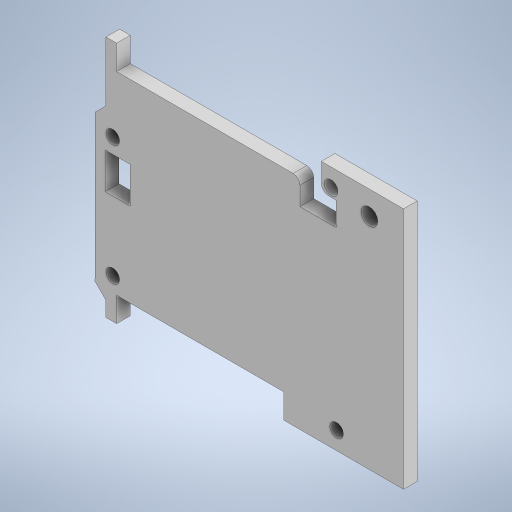
# Autodesk Inventor part: ArduinoCaseTop
Saved by Autodesk Inventor 2024 (Build 280153000, 153)
## iProperties
Created: 2023-09-08
Part Number: ArduinoCaseTop
Material: Generic
Document SubType Name: Modeling
Designer: 18179
Density: 1 g/cm^3
Appearance: Default
Autodesk Inventor part; units mm, degrees
ref_plane "YZ Plane" through (0, 0, 0) normal (1, 0, 0) x (0, 1, 0)
ref_plane "XZ Plane" through (0, 0, 0) normal (0, 1, 0) x (-1, 0, 0)
ref_plane "XY Plane" through (0, 0, 0) normal (0, 0, 1) x (1, 0, 0)
sketch "0" plane through (0, 0, 0) normal (0, 0, 1) x (1, 0, 0)
  line L0 (-4.3025, -38.4925) -> (-4.3025, 26.9125)
  arc A0 (-4.3025, 26.9125) -> (-7.4775, 30.0875) centre (-7.4775, 26.9125) ccw
  line L1 (-7.4775, 30.0875) -> (-8.7475, 30.0875)
  arc A1 (-8.7475, 30.0875) -> (-11.9225, 26.9125) centre (-8.7475, 26.9125) ccw
  line L2 (-11.9225, 26.9125) -> (-11.9225, 22.4675)
  line L3 (-11.9225, 22.4675) -> (-65.8975, 22.4675)
  line L4 (-65.8975, 22.4675) -> (-65.8975, 26.9125)
  arc A2 (-65.8975, 26.9125) -> (-69.0725, 30.0875) centre (-69.0725, 26.9125) ccw
  line L5 (-69.0725, 30.0875) -> (-70.3425, 30.0875)
  arc A3 (-70.3425, 30.0875) -> (-73.5175, 26.9125) centre (-70.3425, 26.9125) ccw
  line L6 (-73.5175, 26.9125) -> (-73.5175, 8.5836)
  line L7 (-73.5175, 8.5836) -> (-76.0575, 6.0436)
  line L8 (-76.0575, 6.0436) -> (-76.0575, -27.38)
  line L9 (-76.0575, -27.38) -> (-76.1056, -27.9894)
  line L10 (-76.1056, -27.9894) -> (-73.5175, -30.5776)
  line L11 (-73.5175, -30.5776) -> (-73.5175, -38.4925)
  arc A4 (-73.5175, -38.4925) -> (-70.3425, -41.6675) centre (-70.3425, -38.4925) ccw
  line L12 (-70.3425, -41.6675) -> (-69.0725, -41.6675)
  arc A5 (-69.0725, -41.6675) -> (-65.8975, -38.4925) centre (-69.0725, -38.4925) ccw
  line L13 (-65.8975, -38.4925) -> (-65.8975, -34.0475)
  line L14 (-65.8975, -34.0475) -> (-11.9225, -34.0475)
  line L15 (-11.9225, -34.0475) -> (-11.9225, -38.4925)
  arc A6 (-11.9225, -38.4925) -> (-8.7475, -41.6675) centre (-8.7475, -38.4925) ccw
  line L16 (-8.7475, -41.6675) -> (-7.4775, -41.6675)
  arc A7 (-7.4775, -41.6675) -> (-4.3025, -38.4925) centre (-7.4775, -38.4925) ccw
  line L17 (-5.89, 20.88) -> (-5.89, -32.46)
  line L18 (-5.89, -32.46) -> (-71.93, -32.46)
  line L19 (-71.93, -32.46) -> (-71.93, -29.92)
  line L20 (-71.93, -29.92) -> (-74.47, -27.38)
  line L21 (-74.47, -27.38) -> (-74.47, 5.386)
  line L22 (-74.47, 5.386) -> (-71.93, 7.926)
  line L23 (-71.93, 7.926) -> (-71.93, 20.88)
  line L24 (-71.93, 20.88) -> (-5.89, 20.88)
  line L25 (-48.816, 17.135) -> (-23.416, 17.135)
  line L26 (-23.416, 17.135) -> (-23.416, 19.545)
  line L27 (-23.416, 19.545) -> (-48.816, 19.545)
  line L28 (-48.816, 19.545) -> (-48.816, 17.135)
  line L29 (-46.546, 19.34) -> (-46.546, 17.34)
  line L30 (-46.546, 17.34) -> (-48.546, 17.34)
  line L31 (-48.546, 17.34) -> (-48.546, 19.34)
  line L32 (-48.546, 19.34) -> (-46.546, 19.34)
  line L33 (-44.006, 19.34) -> (-44.006, 17.34)
  line L34 (-44.006, 17.34) -> (-46.006, 17.34)
  line L35 (-46.006, 17.34) -> (-46.006, 19.34)
  line L36 (-46.006, 19.34) -> (-44.006, 19.34)
  line L37 (-41.466, 19.34) -> (-41.466, 17.34)
  line L38 (-41.466, 17.34) -> (-43.466, 17.34)
  line L39 (-43.466, 17.34) -> (-43.466, 19.34)
  line L40 (-43.466, 19.34) -> (-41.466, 19.34)
  line L41 (-38.926, 19.34) -> (-38.926, 17.34)
  line L42 (-38.926, 17.34) -> (-40.926, 17.34)
  line L43 (-40.926, 17.34) -> (-40.926, 19.34)
  line L44 (-40.926, 19.34) -> (-38.926, 19.34)
  line L45 (-36.386, 19.34) -> (-36.386, 17.34)
  line L46 (-36.386, 17.34) -> (-38.386, 17.34)
  line L47 (-38.386, 17.34) -> (-38.386, 19.34)
  line L48 (-38.386, 19.34) -> (-36.386, 19.34)
  line L49 (-33.846, 19.34) -> (-33.846, 17.34)
  line L50 (-33.846, 17.34) -> (-35.846, 17.34)
  line L51 (-35.846, 17.34) -> (-35.846, 19.34)
  line L52 (-35.846, 19.34) -> (-33.846, 19.34)
  line L53 (-31.306, 19.34) -> (-31.306, 17.34)
  line L54 (-31.306, 17.34) -> (-33.306, 17.34)
  line L55 (-33.306, 17.34) -> (-33.306, 19.34)
  line L56 (-33.306, 19.34) -> (-31.306, 19.34)
  line L57 (-28.766, 19.34) -> (-28.766, 17.34)
  line L58 (-28.766, 17.34) -> (-30.766, 17.34)
  line L59 (-30.766, 17.34) -> (-30.766, 19.34)
  line L60 (-30.766, 19.34) -> (-28.766, 19.34)
  line L61 (-26.226, 17.34) -> (-28.226, 17.34)
  line L62 (-28.226, 17.34) -> (-28.226, 19.34)
  line L63 (-28.226, 19.34) -> (-26.226, 19.34)
  line L64 (-26.226, 19.34) -> (-26.226, 17.34)
  line L65 (-25.686, 17.34) -> (-25.686, 19.34)
  line L66 (-25.686, 19.34) -> (-23.686, 19.34)
  line L67 (-23.686, 19.34) -> (-23.686, 17.34)
  line L68 (-23.686, 17.34) -> (-25.686, 17.34)
  line L69 (-20.87, 16.27) -> (-22.41, 16.27)
  arc A8 (-22.41, 16.27) -> (-22.91, 15.77) centre (-22.41, 15.77) ccw
  arc A9 (-22.91, 15.77) -> (-23.41, 16.27) centre (-23.41, 15.77) ccw
  line L70 (-23.41, 16.27) -> (-24.95, 16.27)
  arc A10 (-24.95, 16.27) -> (-25.45, 15.77) centre (-24.95, 15.77) ccw
  arc A11 (-25.45, 15.77) -> (-25.95, 16.27) centre (-25.95, 15.77) ccw
  line L71 (-25.95, 16.27) -> (-27.49, 16.27)
  arc A12 (-27.49, 16.27) -> (-27.99, 15.77) centre (-27.49, 15.77) ccw
  line L72 (-27.99, 15.77) -> (-27.99, 11.77)
  arc A13 (-27.99, 11.77) -> (-27.49, 11.27) centre (-27.49, 11.77) ccw
  line L73 (-27.49, 11.27) -> (-25.95, 11.27)
  arc A14 (-25.95, 11.27) -> (-25.45, 11.77) centre (-25.95, 11.77) ccw
  arc A15 (-25.45, 11.77) -> (-24.95, 11.27) centre (-24.95, 11.77) ccw
  line L74 (-24.95, 11.27) -> (-23.41, 11.27)
  arc A16 (-23.41, 11.27) -> (-22.91, 11.77) centre (-23.41, 11.77) ccw
  arc A17 (-22.91, 11.77) -> (-22.41, 11.27) centre (-22.41, 11.77) ccw
  line L75 (-22.41, 11.27) -> (-20.87, 11.27)
  arc A18 (-20.87, 11.27) -> (-20.37, 11.77) centre (-20.87, 11.77) ccw
  line L76 (-20.37, 11.77) -> (-20.37, 15.77)
  arc A19 (-20.37, 15.77) -> (-20.87, 16.27) centre (-20.87, 15.77) ccw
  arc A20 (-24.555, 12.6317) -> (-24.555, 12.3643) centre (-24.178, 12.498) ccw
  line L77 (-24.555, 12.6317) -> (-24.555, 12.875)
  line L78 (-24.555, 12.875) -> (-24.3117, 12.875)
  arc A21 (-24.0443, 12.875) -> (-24.3117, 12.875) centre (-24.178, 12.498) ccw
  line L79 (-24.0443, 12.875) -> (-23.805, 12.875)
  line L80 (-23.805, 12.875) -> (-23.805, 12.6425)
  arc A22 (-23.805, 12.3535) -> (-23.805, 12.6425) centre (-24.178, 12.498) ccw
  line L81 (-23.805, 12.3535) -> (-23.805, 12.125)
  line L82 (-23.805, 12.125) -> (-24.0335, 12.125)
  arc A23 (-24.3225, 12.125) -> (-24.0335, 12.125) centre (-24.178, 12.498) ccw
  line L83 (-24.3225, 12.125) -> (-24.555, 12.125)
  line L84 (-24.555, 12.125) -> (-24.555, 12.3643)
  arc A24 (-24.555, 15.1717) -> (-24.555, 14.9043) centre (-24.178, 15.038) ccw
  line L85 (-24.555, 15.1717) -> (-24.555, 15.415)
  line L86 (-24.555, 15.415) -> (-24.3117, 15.415)
  arc A25 (-24.0443, 15.415) -> (-24.3117, 15.415) centre (-24.178, 15.038) ccw
  line L87 (-24.0443, 15.415) -> (-23.805, 15.415)
  line L88 (-23.805, 15.415) -> (-23.805, 15.1825)
  arc A26 (-23.805, 14.8935) -> (-23.805, 15.1825) centre (-24.178, 15.038) ccw
  line L89 (-23.805, 14.8935) -> (-23.805, 14.665)
  line L90 (-23.805, 14.665) -> (-24.0335, 14.665)
  arc A27 (-24.3225, 14.665) -> (-24.0335, 14.665) centre (-24.178, 15.038) ccw
  line L91 (-24.3225, 14.665) -> (-24.555, 14.665)
  line L92 (-24.555, 14.665) -> (-24.555, 14.9043)
  arc A28 (-27.095, 12.6317) -> (-27.095, 12.3643) centre (-26.718, 12.498) ccw
  line L93 (-27.095, 12.6317) -> (-27.095, 12.875)
  line L94 (-27.095, 12.875) -> (-26.8517, 12.875)
  arc A29 (-26.5843, 12.875) -> (-26.8517, 12.875) centre (-26.718, 12.498) ccw
  line L95 (-26.5843, 12.875) -> (-26.345, 12.875)
  line L96 (-26.345, 12.875) -> (-26.345, 12.6425)
  arc A30 (-26.345, 12.3535) -> (-26.345, 12.6425) centre (-26.718, 12.498) ccw
  line L97 (-26.345, 12.3535) -> (-26.345, 12.125)
  line L98 (-26.345, 12.125) -> (-26.5735, 12.125)
  arc A31 (-26.8625, 12.125) -> (-26.5735, 12.125) centre (-26.718, 12.498) ccw
  line L99 (-26.8625, 12.125) -> (-27.095, 12.125)
  line L100 (-27.095, 12.125) -> (-27.095, 12.3643)
  arc A32 (-27.095, 15.1717) -> (-27.095, 14.9043) centre (-26.718, 15.038) ccw
  line L101 (-27.095, 15.1717) -> (-27.095, 15.415)
  line L102 (-27.095, 15.415) -> (-26.8517, 15.415)
  arc A33 (-26.5843, 15.415) -> (-26.8517, 15.415) centre (-26.718, 15.038) ccw
  line L103 (-26.5843, 15.415) -> (-26.345, 15.415)
  line L104 (-26.345, 15.415) -> (-26.345, 15.1825)
  arc A34 (-26.345, 14.8935) -> (-26.345, 15.1825) centre (-26.718, 15.038) ccw
  line L105 (-26.345, 14.8935) -> (-26.345, 14.665)
  line L106 (-26.345, 14.665) -> (-26.5735, 14.665)
  arc A35 (-26.8625, 14.665) -> (-26.5735, 14.665) centre (-26.718, 15.038) ccw
  line L107 (-26.8625, 14.665) -> (-27.095, 14.665)
  line L108 (-27.095, 14.665) -> (-27.095, 14.9043)
  arc A36 (-22.015, 12.6317) -> (-22.015, 12.3643) centre (-21.638, 12.498) ccw
  line L109 (-22.015, 12.6317) -> (-22.015, 12.875)
  line L110 (-22.015, 12.875) -> (-21.7717, 12.875)
  arc A37 (-21.5043, 12.875) -> (-21.7717, 12.875) centre (-21.638, 12.498) ccw
  line L111 (-21.5043, 12.875) -> (-21.265, 12.875)
  line L112 (-21.265, 12.875) -> (-21.265, 12.6425)
  arc A38 (-21.265, 12.3535) -> (-21.265, 12.6425) centre (-21.638, 12.498) ccw
  line L113 (-21.265, 12.3535) -> (-21.265, 12.125)
  line L114 (-21.265, 12.125) -> (-21.4935, 12.125)
  arc A39 (-21.7825, 12.125) -> (-21.4935, 12.125) centre (-21.638, 12.498) ccw
  line L115 (-21.7825, 12.125) -> (-22.015, 12.125)
  line L116 (-22.015, 12.125) -> (-22.015, 12.3643)
  arc A40 (-22.015, 15.1717) -> (-22.015, 14.9043) centre (-21.638, 15.038) ccw
  line L117 (-22.015, 15.1717) -> (-22.015, 15.415)
  line L118 (-22.015, 15.415) -> (-21.7717, 15.415)
  arc A41 (-21.5043, 15.415) -> (-21.7717, 15.415) centre (-21.638, 15.038) ccw
  line L119 (-21.5043, 15.415) -> (-21.265, 15.415)
  line L120 (-21.265, 15.415) -> (-21.265, 15.1825)
  arc A42 (-21.265, 14.8935) -> (-21.265, 15.1825) centre (-21.638, 15.038) ccw
  line L121 (-21.265, 14.8935) -> (-21.265, 14.665)
  line L122 (-21.265, 14.665) -> (-21.4935, 14.665)
  arc A43 (-21.7825, 14.665) -> (-21.4935, 14.665) centre (-21.638, 15.038) ccw
  line L123 (-21.7825, 14.665) -> (-22.015, 14.665)
  line L124 (-22.015, 14.665) -> (-22.015, 14.9043)
  line L125 (-70.66, 17.135) -> (-50.34, 17.135)
  line L126 (-50.34, 17.135) -> (-50.34, 19.545)
  line L127 (-50.34, 19.545) -> (-70.66, 19.545)
  line L128 (-70.66, 19.545) -> (-70.66, 17.135)
  line L129 (-68.39, 19.34) -> (-68.39, 17.34)
  line L130 (-68.39, 17.34) -> (-70.39, 17.34)
  line L131 (-70.39, 17.34) -> (-70.39, 19.34)
  line L132 (-70.39, 19.34) -> (-68.39, 19.34)
  line L133 (-65.85, 19.34) -> (-65.85, 17.34)
  line L134 (-65.85, 17.34) -> (-67.85, 17.34)
  line L135 (-67.85, 17.34) -> (-67.85, 19.34)
  line L136 (-67.85, 19.34) -> (-65.85, 19.34)
  line L137 (-63.31, 19.34) -> (-63.31, 17.34)
  line L138 (-63.31, 17.34) -> (-65.31, 17.34)
  line L139 (-65.31, 17.34) -> (-65.31, 19.34)
  line L140 (-65.31, 19.34) -> (-63.31, 19.34)
  line L141 (-60.77, 19.34) -> (-60.77, 17.34)
  line L142 (-60.77, 17.34) -> (-62.77, 17.34)
  line L143 (-62.77, 17.34) -> (-62.77, 19.34)
  line L144 (-62.77, 19.34) -> (-60.77, 19.34)
  line L145 (-58.23, 19.34) -> (-58.23, 17.34)
  line L146 (-58.23, 17.34) -> (-60.23, 17.34)
  line L147 (-60.23, 17.34) -> (-60.23, 19.34)
  line L148 (-60.23, 19.34) -> (-58.23, 19.34)
  line L149 (-55.69, 19.34) -> (-55.69, 17.34)
  line L150 (-55.69, 17.34) -> (-57.69, 17.34)
  line L151 (-57.69, 17.34) -> (-57.69, 19.34)
  line L152 (-57.69, 19.34) -> (-55.69, 19.34)
  line L153 (-53.15, 17.34) -> (-55.15, 17.34)
  line L154 (-55.15, 17.34) -> (-55.15, 19.34)
  line L155 (-55.15, 19.34) -> (-53.15, 19.34)
  line L156 (-53.15, 19.34) -> (-53.15, 17.34)
  line L157 (-52.61, 17.34) -> (-52.61, 19.34)
  line L158 (-52.61, 19.34) -> (-50.61, 19.34)
  line L159 (-50.61, 19.34) -> (-50.61, 17.34)
  line L160 (-50.61, 17.34) -> (-52.61, 17.34)
  line L161 (-73.3, -1.26) -> (-73.3, -2.8)
  arc A44 (-73.3, -2.8) -> (-72.8, -3.3) centre (-72.8, -2.8) ccw
  arc A45 (-72.8, -3.3) -> (-73.3, -3.8) centre (-72.8, -3.8) ccw
  line L162 (-73.3, -3.8) -> (-73.3, -5.34)
  arc A46 (-73.3, -5.34) -> (-72.8, -5.84) centre (-72.8, -5.34) ccw
  arc A47 (-72.8, -5.84) -> (-73.3, -6.34) centre (-72.8, -6.34) ccw
  line L163 (-73.3, -6.34) -> (-73.3, -7.88)
  arc A48 (-73.3, -7.88) -> (-72.8, -8.38) centre (-72.8, -7.88) ccw
  line L164 (-72.8, -8.38) -> (-68.8, -8.38)
  arc A49 (-68.8, -8.38) -> (-68.3, -7.88) centre (-68.8, -7.88) ccw
  line L165 (-68.3, -7.88) -> (-68.3, -6.34)
  arc A50 (-68.3, -6.34) -> (-68.8, -5.84) centre (-68.8, -6.34) ccw
  arc A51 (-68.8, -5.84) -> (-68.3, -5.34) centre (-68.8, -5.34) ccw
  line L166 (-68.3, -5.34) -> (-68.3, -3.8)
  arc A52 (-68.3, -3.8) -> (-68.8, -3.3) centre (-68.8, -3.8) ccw
  arc A53 (-68.8, -3.3) -> (-68.3, -2.8) centre (-68.8, -2.8) ccw
  line L167 (-68.3, -2.8) -> (-68.3, -1.26)
  arc A54 (-68.3, -1.26) -> (-68.8, -0.76) centre (-68.8, -1.26) ccw
  line L168 (-68.8, -0.76) -> (-72.8, -0.76)
  arc A55 (-72.8, -0.76) -> (-73.3, -1.26) centre (-72.8, -1.26) ccw
  arc A56 (-69.905, -4.4308) -> (-69.905, -4.7092) centre (-69.53, -4.57) ccw
  line L169 (-69.905, -4.4308) -> (-69.905, -4.195)
  line L170 (-69.905, -4.195) -> (-69.6692, -4.195)
  arc A57 (-69.3908, -4.195) -> (-69.6692, -4.195) centre (-69.53, -4.57) ccw
  line L171 (-69.3908, -4.195) -> (-69.155, -4.195)
  line L172 (-69.155, -4.195) -> (-69.155, -4.4308)
  arc A58 (-69.155, -4.7092) -> (-69.155, -4.4308) centre (-69.53, -4.57) ccw
  line L173 (-69.155, -4.7092) -> (-69.155, -4.945)
  line L174 (-69.155, -4.945) -> (-69.3908, -4.945)
  arc A59 (-69.6692, -4.945) -> (-69.3908, -4.945) centre (-69.53, -4.57) ccw
  line L175 (-69.6692, -4.945) -> (-69.905, -4.945)
  line L176 (-69.905, -4.945) -> (-69.905, -4.7092)
  arc A60 (-72.445, -4.4308) -> (-72.445, -4.7092) centre (-72.07, -4.57) ccw
  line L177 (-72.445, -4.4308) -> (-72.445, -4.195)
  line L178 (-72.445, -4.195) -> (-72.2092, -4.195)
  arc A61 (-71.9308, -4.195) -> (-72.2092, -4.195) centre (-72.07, -4.57) ccw
  line L179 (-71.9308, -4.195) -> (-71.695, -4.195)
  line L180 (-71.695, -4.195) -> (-71.695, -4.4308)
  arc A62 (-71.695, -4.7092) -> (-71.695, -4.4308) centre (-72.07, -4.57) ccw
  line L181 (-71.695, -4.7092) -> (-71.695, -4.945)
  line L182 (-71.695, -4.945) -> (-71.9308, -4.945)
  arc A63 (-72.2092, -4.945) -> (-71.9308, -4.945) centre (-72.07, -4.57) ccw
  line L183 (-72.2092, -4.945) -> (-72.445, -4.945)
  line L184 (-72.445, -4.945) -> (-72.445, -4.7092)
  arc A64 (-69.905, -6.9708) -> (-69.905, -7.2492) centre (-69.53, -7.11) ccw
  line L185 (-69.905, -6.9708) -> (-69.905, -6.735)
  line L186 (-69.905, -6.735) -> (-69.6692, -6.735)
  arc A65 (-69.3908, -6.735) -> (-69.6692, -6.735) centre (-69.53, -7.11) ccw
  line L187 (-69.3908, -6.735) -> (-69.155, -6.735)
  line L188 (-69.155, -6.735) -> (-69.155, -6.9708)
  arc A66 (-69.155, -7.2492) -> (-69.155, -6.9708) centre (-69.53, -7.11) ccw
  line L189 (-69.155, -7.2492) -> (-69.155, -7.485)
  line L190 (-69.155, -7.485) -> (-69.3908, -7.485)
  arc A67 (-69.6692, -7.485) -> (-69.3908, -7.485) centre (-69.53, -7.11) ccw
  line L191 (-69.6692, -7.485) -> (-69.905, -7.485)
  line L192 (-69.905, -7.485) -> (-69.905, -7.2492)
  line L193 (-72.445, -7.485) -> (-72.445, -6.735)
  line L194 (-72.445, -6.735) -> (-71.695, -6.735)
  line L195 (-71.695, -6.735) -> (-71.695, -7.485)
  line L196 (-71.695, -7.485) -> (-72.445, -7.485)
  arc A68 (-69.905, -1.8908) -> (-69.905, -2.1692) centre (-69.53, -2.03) ccw
  line L197 (-69.905, -1.8908) -> (-69.905, -1.655)
  line L198 (-69.905, -1.655) -> (-69.6692, -1.655)
  arc A69 (-69.3908, -1.655) -> (-69.6692, -1.655) centre (-69.53, -2.03) ccw
  line L199 (-69.3908, -1.655) -> (-69.155, -1.655)
  line L200 (-69.155, -1.655) -> (-69.155, -1.8908)
  arc A70 (-69.155, -2.1692) -> (-69.155, -1.8908) centre (-69.53, -2.03) ccw
  line L201 (-69.155, -2.1692) -> (-69.155, -2.405)
  line L202 (-69.155, -2.405) -> (-69.3908, -2.405)
  arc A71 (-69.6692, -2.405) -> (-69.3908, -2.405) centre (-69.53, -2.03) ccw
  line L203 (-69.6692, -2.405) -> (-69.905, -2.405)
  line L204 (-69.905, -2.405) -> (-69.905, -2.1692)
  arc A72 (-72.445, -1.8908) -> (-72.445, -2.1692) centre (-72.07, -2.03) ccw
  line L205 (-72.445, -1.8908) -> (-72.445, -1.655)
  line L206 (-72.445, -1.655) -> (-72.2092, -1.655)
  arc A73 (-71.9308, -1.655) -> (-72.2092, -1.655) centre (-72.07, -2.03) ccw
  line L207 (-71.9308, -1.655) -> (-71.695, -1.655)
  line L208 (-71.695, -1.655) -> (-71.695, -1.8908)
  arc A74 (-71.695, -2.1692) -> (-71.695, -1.8908) centre (-72.07, -2.03) ccw
  line L209 (-71.695, -2.1692) -> (-71.695, -2.405)
  line L210 (-71.695, -2.405) -> (-71.9308, -2.405)
  arc A75 (-72.2092, -2.405) -> (-71.9308, -2.405) centre (-72.07, -2.03) ccw
  line L211 (-72.2092, -2.405) -> (-72.445, -2.405)
  line L212 (-72.445, -2.405) -> (-72.445, -2.1692)
  line L213 (-70.66, -31.125) -> (-55.42, -31.125)
  line L214 (-55.42, -31.125) -> (-55.42, -28.715)
  line L215 (-55.42, -28.715) -> (-70.66, -28.715)
  line L216 (-70.66, -28.715) -> (-70.66, -31.125)
  line L217 (-68.39, -28.92) -> (-68.39, -30.92)
  line L218 (-68.39, -30.92) -> (-70.39, -30.92)
  line L219 (-70.39, -30.92) -> (-70.39, -28.92)
  line L220 (-70.39, -28.92) -> (-68.39, -28.92)
  line L221 (-65.85, -28.92) -> (-65.85, -30.92)
  line L222 (-65.85, -30.92) -> (-67.85, -30.92)
  line L223 (-67.85, -30.92) -> (-67.85, -28.92)
  line L224 (-67.85, -28.92) -> (-65.85, -28.92)
  line L225 (-63.31, -28.92) -> (-63.31, -30.92)
  line L226 (-63.31, -30.92) -> (-65.31, -30.92)
  line L227 (-65.31, -30.92) -> (-65.31, -28.92)
  line L228 (-65.31, -28.92) -> (-63.31, -28.92)
  line L229 (-60.77, -28.92) -> (-60.77, -30.92)
  line L230 (-60.77, -30.92) -> (-62.77, -30.92)
  line L231 (-62.77, -30.92) -> (-62.77, -28.92)
  line L232 (-62.77, -28.92) -> (-60.77, -28.92)
  line L233 (-58.23, -30.92) -> (-60.23, -30.92)
  line L234 (-60.23, -30.92) -> (-60.23, -28.92)
  line L235 (-60.23, -28.92) -> (-58.23, -28.92)
  line L236 (-58.23, -28.92) -> (-58.23, -30.92)
  line L237 (-57.69, -30.92) -> (-57.69, -28.92)
  line L238 (-57.69, -28.92) -> (-55.69, -28.92)
  line L239 (-55.69, -28.92) -> (-55.69, -30.92)
  line L240 (-55.69, -30.92) -> (-57.69, -30.92)
  line L241 (-52.88, -31.125) -> (-32.56, -31.125)
  line L242 (-32.56, -31.125) -> (-32.56, -28.715)
  line L243 (-32.56, -28.715) -> (-52.88, -28.715)
  line L244 (-52.88, -28.715) -> (-52.88, -31.125)
  line L245 (-50.61, -28.92) -> (-50.61, -30.92)
  line L246 (-50.61, -30.92) -> (-52.61, -30.92)
  line L247 (-52.61, -30.92) -> (-52.61, -28.92)
  line L248 (-52.61, -28.92) -> (-50.61, -28.92)
  line L249 (-48.07, -28.92) -> (-48.07, -30.92)
  line L250 (-48.07, -30.92) -> (-50.07, -30.92)
  line L251 (-50.07, -30.92) -> (-50.07, -28.92)
  line L252 (-50.07, -28.92) -> (-48.07, -28.92)
  line L253 (-45.53, -28.92) -> (-45.53, -30.92)
  line L254 (-45.53, -30.92) -> (-47.53, -30.92)
  line L255 (-47.53, -30.92) -> (-47.53, -28.92)
  line L256 (-47.53, -28.92) -> (-45.53, -28.92)
  line L257 (-42.99, -28.92) -> (-42.99, -30.92)
  line L258 (-42.99, -30.92) -> (-44.99, -30.92)
  line L259 (-44.99, -30.92) -> (-44.99, -28.92)
  line L260 (-44.99, -28.92) -> (-42.99, -28.92)
  line L261 (-40.45, -28.92) -> (-40.45, -30.92)
  line L262 (-40.45, -30.92) -> (-42.45, -30.92)
  line L263 (-42.45, -30.92) -> (-42.45, -28.92)
  line L264 (-42.45, -28.92) -> (-40.45, -28.92)
  line L265 (-37.91, -28.92) -> (-37.91, -30.92)
  line L266 (-37.91, -30.92) -> (-39.91, -30.92)
  line L267 (-39.91, -30.92) -> (-39.91, -28.92)
  line L268 (-39.91, -28.92) -> (-37.91, -28.92)
  line L269 (-35.37, -30.92) -> (-37.37, -30.92)
  line L270 (-37.37, -30.92) -> (-37.37, -28.92)
  line L271 (-37.37, -28.92) -> (-35.37, -28.92)
  line L272 (-35.37, -28.92) -> (-35.37, -30.92)
  line L273 (-34.83, -30.92) -> (-34.83, -28.92)
  line L274 (-34.83, -28.92) -> (-32.83, -28.92)
  line L275 (-32.83, -28.92) -> (-32.83, -30.92)
  line L276 (-32.83, -30.92) -> (-34.83, -30.92)
  line L277 (-74.5335, 0.814) -> (-71.93, 0.814)
  arc A76 (-71.93, 0.814) -> (-71.93, 5.386) centre (-71.93, 3.1) ccw
  line L278 (-71.93, 5.386) -> (-74.5335, 5.386)
  line L279 (-74.5335, 5.386) -> (-74.5335, 5.4123)
  line L280 (-74.5335, 5.4123) -> (-71.9935, 7.9523)
  line L281 (-71.9935, 7.9523) -> (-71.9935, 20.9435)
  line L282 (-71.9935, 20.9435) -> (-23.416, 20.9435)
  line L283 (-23.416, 20.9435) -> (-23.416, 18.34)
  arc A77 (-23.416, 18.34) -> (-18.844, 18.34) centre (-21.13, 18.34) ccw
  line L284 (-18.844, 18.34) -> (-18.844, 20.9435)
  line L285 (-18.844, 20.9435) -> (-5.8265, 20.9435)
  line L286 (-5.8265, 20.9435) -> (-5.8265, 11.12)
  line L287 (-5.8265, 11.12) -> (-5.89, 11.12)
  line L288 (-5.89, 11.12) -> (-5.89, 0)
  line L289 (-5.89, 0) -> (-5.8265, 0)
  line L290 (-5.8265, 0) -> (-5.8265, -20.285)
  line L291 (-5.8265, -20.285) -> (-5.89, -20.285)
  line L292 (-5.89, -20.285) -> (-5.89, -29.285)
  line L293 (-5.89, -29.285) -> (-5.8265, -29.285)
  line L294 (-5.8265, -29.285) -> (-5.8265, -32.5235)
  line L295 (-5.8265, -32.5235) -> (-71.9935, -32.5235)
  line L296 (-71.9935, -32.5235) -> (-71.9935, -29.9463)
  line L297 (-71.9935, -29.9463) -> (-74.5335, -27.4063)
  line L298 (-74.5335, -27.4063) -> (-74.5335, -27.126)
  line L299 (-74.5335, -27.126) -> (-71.93, -27.126)
  arc A78 (-71.93, -27.126) -> (-71.93, -22.554) centre (-71.93, -24.84) ccw
  line L300 (-71.93, -22.554) -> (-74.5335, -22.554)
  line L301 (-74.5335, -22.554) -> (-74.5335, 0.814)
  line L302 (-22.146, -29.92) -> (-22.146, -32.46)
  line L303 (-22.146, -32.46) -> (-17.574, -32.46)
  line L304 (-17.574, -32.46) -> (-17.574, -29.92)
  arc A79 (-17.574, -29.92) -> (-22.146, -29.92) centre (-19.86, -29.92) ccw
  circle A80 centre (-8.1125, -37.8575) radius 2
  circle A81 centre (-69.7075, -37.8575) radius 2
  circle A82 centre (-69.7075, 26.2775) radius 2
  circle A83 centre (-8.1125, 26.2775) radius 2
  line L305 (-47.53, -28.92) -> (-47.53, -30.92)
  circle A84 centre (-12.24, 16.943) radius 1.5
  point P0 (-20.37, 11.77)
  point P1 (-22.41, 11.27)
  point P2 (-22.91, 11.77)
  point P3 (-24.95, 11.27)
  point P4 (-27.99, 15.77)
  point P5 (-23.41, 16.27)
  point P6 (-22.91, 15.77)
  point P7 (-68.8, -0.76)
  point P8 (-68.8, -5.84)
  point P9 (-72.8, -8.38)
  point P10 (-73.5175, 26.9125)
  point P11 (-11.9225, -34.0475)
  point P12 (-74.47, 0.814)
  point P13 (-23.416, 20.88)
  point P14 (-18.844, 20.88)
  point P15 (-18.844, 18.34)
  point P16 (-20.528, 16.1347)
  point P17 (-22.1, 16.27)
  point P18 (-74.47, -27.126)
  point P19 (-74.47, -22.554)
  constraints: 612 end point, 160 point on circle, 85 centre point
extrude "Extrusion1" add sketch "0" along normal blind 3.175 contours A7 L16 A6 L15 L14 L13 A5 L12 A4 L11 L10 L9 L8 L7 L6 A3 L5 A2 L4 L3 L2 A1 L1 A0 L0 | L24 L284 L285 L286 L287 L17 | L17 L18 L304 A79 L302 L19 L20 L21 L299 A78 L300 L277 A76 L278 L22 L23 L24 L283 L27 L28 L25 L26 A77 L69 A8 A9 L70 A10 A11 L71 A12 L72 A13 L73 A14 A15 L74 A16 A17 L75 A18 L76 A19 L284 | L289 L290 L291 L17 | L24 L23 L22 L278 L279 L280 L281 L282 L283 | L293 L294 L295 L296 L297 L298 L299 L21 L20 L19 L18 L17 | L21 L300 L301 L277
sketch "Sketch3" plane through (0, 0, 3.175) normal (0, 0, 1) x (1, 0, 0)
  line L0 (-11.9225, 22.4675) -> (-65.8975, 22.4675) projected
  line L1 (-65.8975, 22.4675) -> (-76.7323, 22.4675)
  line L2 (-76.7323, 22.4675) -> (-76.7323, 33.3993)
  line L3 (-76.7323, 33.3993) -> (-65.8975, 33.3993)
  line L4 (-65.8975, 33.3993) -> (-65.8975, 22.4675)
  line L5 (-11.9225, 22.4675) -> (0, 22.4675)
  line L6 (0, 22.4675) -> (0, 30.8652)
  line L7 (0, 30.8652) -> (-11.9225, 30.8652)
  line L8 (-11.9225, 30.8652) -> (-11.9225, 22.4675)
  line L9 (-65.8975, -34.0475) -> (-11.9225, -34.0475) projected
  line L10 (-11.9225, -34.0475) -> (4.7641, -34.0475)
  line L11 (4.7641, -34.0475) -> (4.7641, -42.8261)
  line L12 (4.7641, -42.8261) -> (-11.9225, -42.8261)
  line L13 (-11.9225, -42.8261) -> (-11.9225, -34.0475)
  line L14 (-65.8975, -34.0475) -> (-80.7868, -34.0475)
  line L15 (-80.7868, -34.0475) -> (-80.7868, -44.3466)
  line L16 (-80.7868, -44.3466) -> (-65.8975, -44.3466)
  line L17 (-65.8975, -44.3466) -> (-65.8975, -34.0475)
  line L18 (-68.3, -8.38) -> (-73.3, -8.38)
  line L19 (-73.3, -8.38) -> (-73.3, -0.76)
  line L20 (-73.3, -0.76) -> (-68.3, -0.76)
  line L21 (-68.3, -0.76) -> (-68.3, -8.38)
  line L22 (-27.99, 16.27) -> (-20.37, 16.27)
  line L23 (-20.37, 16.27) -> (-20.37, 11.27)
  line L24 (-20.37, 11.27) -> (-27.99, 11.27)
  line L25 (-27.99, 11.27) -> (-27.99, 16.27)
  arc A0 (-4.3025, 26.9125) -> (-7.4775, 30.0875) centre (-7.4775, 26.9125) ccw projected
  line L26 (-7.4775, 30.0875) -> (-8.7475, 30.0875) projected
  arc A1 (-8.7475, 30.0875) -> (-11.9225, 26.9125) centre (-8.7475, 26.9125) ccw projected
  line L27 (-11.9225, 26.9125) -> (-11.9225, 22.4675) projected
  line L28 (-11.9225, 22.4675) -> (-65.8975, 22.4675) projected
  line L29 (-65.8975, 22.4675) -> (-65.8975, 26.9125) projected
  arc A2 (-65.8975, 26.9125) -> (-69.0725, 30.0875) centre (-69.0725, 26.9125) ccw projected
  line L30 (-69.0725, 30.0875) -> (-70.3425, 30.0875) projected
  arc A3 (-70.3425, 30.0875) -> (-73.5175, 26.9125) centre (-70.3425, 26.9125) ccw projected
  line L31 (-73.5175, 26.9125) -> (-73.5175, 8.5836) projected
  line L32 (-73.5175, 8.5836) -> (-76.0575, 6.0436) projected
  line L33 (-76.0575, 6.0436) -> (-76.0575, -27.38) projected
  line L34 (-76.0575, -27.38) -> (-76.1056, -27.9894) projected
  line L35 (-76.1056, -27.9894) -> (-73.5175, -30.5776) projected
  line L36 (-73.5175, -30.5776) -> (-73.5175, -38.4925) projected
  arc A4 (-73.5175, -38.4925) -> (-70.3425, -41.6675) centre (-70.3425, -38.4925) ccw projected
  line L37 (-70.3425, -41.6675) -> (-69.0725, -41.6675) projected
  arc A5 (-69.0725, -41.6675) -> (-65.8975, -38.4925) centre (-69.0725, -38.4925) ccw projected
  line L38 (-65.8975, -38.4925) -> (-65.8975, -34.0475) projected
  line L39 (-65.8975, -34.0475) -> (-11.9225, -34.0475) projected
  line L40 (-11.9225, -34.0475) -> (-11.9225, -38.4925) projected
  arc A6 (-11.9225, -38.4925) -> (-8.7475, -41.6675) centre (-8.7475, -38.4925) ccw projected
  line L41 (-8.7475, -41.6675) -> (-7.4775, -41.6675) projected
  arc A7 (-7.4775, -41.6675) -> (-4.3025, -38.4925) centre (-7.4775, -38.4925) ccw projected
  line L42 (-4.3025, -38.4925) -> (-4.3025, 26.9125) projected
  line L43 (-23.416, 18.34) -> (-23.416, 17.135) projected
  line L44 (-23.416, 17.135) -> (-48.816, 17.135) projected
  line L45 (-48.816, 17.135) -> (-48.816, 19.545) projected
  line L46 (-48.816, 19.545) -> (-23.416, 19.545) projected
  line L47 (-22.41, 16.27) -> (-22.1, 16.27) projected
  arc A8 (-20.37, 15.77) -> (-20.528, 16.1347) centre (-20.87, 15.77) ccw projected
  line L48 (-20.37, 15.77) -> (-20.37, 11.77) projected
  arc A9 (-20.87, 11.27) -> (-20.37, 11.77) centre (-20.87, 11.77) ccw projected
  line L49 (-20.87, 11.27) -> (-22.41, 11.27) projected
  arc A10 (-22.91, 11.77) -> (-22.41, 11.27) centre (-22.41, 11.77) ccw projected
  arc A11 (-23.41, 11.27) -> (-22.91, 11.77) centre (-23.41, 11.77) ccw projected
  line L50 (-23.41, 11.27) -> (-24.95, 11.27) projected
  arc A12 (-25.45, 11.77) -> (-24.95, 11.27) centre (-24.95, 11.77) ccw projected
  arc A13 (-25.95, 11.27) -> (-25.45, 11.77) centre (-25.95, 11.77) ccw projected
  line L51 (-25.95, 11.27) -> (-27.49, 11.27) projected
  arc A14 (-27.99, 11.77) -> (-27.49, 11.27) centre (-27.49, 11.77) ccw projected
  line L52 (-27.99, 11.77) -> (-27.99, 15.77) projected
  arc A15 (-27.49, 16.27) -> (-27.99, 15.77) centre (-27.49, 15.77) ccw projected
  line L53 (-27.49, 16.27) -> (-25.95, 16.27) projected
  arc A16 (-25.45, 15.77) -> (-25.95, 16.27) centre (-25.95, 15.77) ccw projected
  arc A17 (-24.95, 16.27) -> (-25.45, 15.77) centre (-24.95, 15.77) ccw projected
  line L54 (-24.95, 16.27) -> (-23.41, 16.27) projected
  arc A18 (-22.91, 15.77) -> (-23.41, 16.27) centre (-23.41, 15.77) ccw projected
  arc A19 (-22.41, 16.27) -> (-22.91, 15.77) centre (-22.41, 15.77) ccw projected
  line L55 (-70.66, 17.135) -> (-70.66, 19.545) projected
  line L56 (-70.66, 19.545) -> (-50.34, 19.545) projected
  line L57 (-50.34, 19.545) -> (-50.34, 17.135) projected
  line L58 (-50.34, 17.135) -> (-70.66, 17.135) projected
  arc A20 (-72.8, -0.76) -> (-73.3, -1.26) centre (-72.8, -1.26) ccw projected
  line L59 (-72.8, -0.76) -> (-68.8, -0.76) projected
  arc A21 (-68.3, -1.26) -> (-68.8, -0.76) centre (-68.8, -1.26) ccw projected
  line L60 (-68.3, -1.26) -> (-68.3, -2.8) projected
  arc A22 (-68.8, -3.3) -> (-68.3, -2.8) centre (-68.8, -2.8) ccw projected
  arc A23 (-68.3, -3.8) -> (-68.8, -3.3) centre (-68.8, -3.8) ccw projected
  line L61 (-68.3, -3.8) -> (-68.3, -5.34) projected
  arc A24 (-68.8, -5.84) -> (-68.3, -5.34) centre (-68.8, -5.34) ccw projected
  arc A25 (-68.3, -6.34) -> (-68.8, -5.84) centre (-68.8, -6.34) ccw projected
  line L62 (-68.3, -6.34) -> (-68.3, -7.88) projected
  arc A26 (-68.8, -8.38) -> (-68.3, -7.88) centre (-68.8, -7.88) ccw projected
  line L63 (-68.8, -8.38) -> (-72.8, -8.38) projected
  arc A27 (-73.3, -7.88) -> (-72.8, -8.38) centre (-72.8, -7.88) ccw projected
  line L64 (-73.3, -7.88) -> (-73.3, -6.34) projected
  arc A28 (-72.8, -5.84) -> (-73.3, -6.34) centre (-72.8, -6.34) ccw projected
  arc A29 (-73.3, -5.34) -> (-72.8, -5.84) centre (-72.8, -5.34) ccw projected
  line L65 (-73.3, -5.34) -> (-73.3, -3.8) projected
  arc A30 (-72.8, -3.3) -> (-73.3, -3.8) centre (-72.8, -3.8) ccw projected
  arc A31 (-73.3, -2.8) -> (-72.8, -3.3) centre (-72.8, -2.8) ccw projected
  line L66 (-73.3, -2.8) -> (-73.3, -1.26) projected
  line L67 (-70.66, -31.125) -> (-70.66, -28.715) projected
  line L68 (-70.66, -28.715) -> (-55.42, -28.715) projected
  line L69 (-55.42, -28.715) -> (-55.42, -31.125) projected
  line L70 (-55.42, -31.125) -> (-70.66, -31.125) projected
  line L71 (-52.88, -31.125) -> (-52.88, -28.715) projected
  line L72 (-52.88, -28.715) -> (-32.56, -28.715) projected
  line L73 (-32.56, -28.715) -> (-32.56, -31.125) projected
  line L74 (-32.56, -31.125) -> (-52.88, -31.125) projected
  circle A32 centre (-12.24, 16.943) radius 1.5 projected
  circle A33 centre (-8.1125, 26.2775) radius 2 projected
  circle A34 centre (-69.7075, 26.2775) radius 2 projected
  circle A35 centre (-69.7075, -37.8575) radius 2 projected
  circle A36 centre (-8.1125, -37.8575) radius 2 projected
  line L75 (-28.371, 10.889) -> (-19.989, 10.889)
  line L76 (-19.989, 10.889) -> (-19.989, 16.651)
  line L77 (-19.989, 16.651) -> (-28.371, 16.651)
  line L78 (-28.371, 16.651) -> (-28.371, 10.889)
  line L79 (-49.197, 16.754) -> (-23.035, 16.754)
  line L80 (-23.035, 16.754) -> (-23.035, 19.926)
  line L81 (-23.035, 19.926) -> (-49.197, 19.926)
  line L82 (-49.197, 19.926) -> (-49.197, 16.754)
  line L83 (-71.041, 16.754) -> (-71.041, 19.926)
  line L84 (-71.041, 19.926) -> (-49.959, 19.926)
  line L85 (-49.959, 19.926) -> (-49.959, 16.754)
  line L86 (-49.959, 16.754) -> (-71.041, 16.754)
  line L87 (-67.919, -8.761) -> (-73.681, -8.761)
  line L88 (-73.681, -8.761) -> (-73.681, -0.379)
  line L89 (-73.681, -0.379) -> (-67.919, -0.379)
  line L90 (-67.919, -0.379) -> (-67.919, -8.761)
  line L91 (-55.039, -28.334) -> (-71.041, -28.334)
  line L92 (-71.041, -28.334) -> (-71.041, -31.506)
  line L93 (-71.041, -31.506) -> (-55.039, -31.506)
  line L94 (-55.039, -31.506) -> (-55.039, -28.334)
  line L95 (-32.179, -28.334) -> (-53.261, -28.334)
  line L96 (-53.261, -28.334) -> (-53.261, -31.506)
  line L97 (-53.261, -31.506) -> (-32.179, -31.506)
  line L98 (-32.179, -31.506) -> (-32.179, -28.334)
  circle A37 centre (-12.24, 16.943) radius 1.627
  line L99 (-23.416, 20.88) -> (-18.844, 20.88) projected
  line L100 (-18.844, 20.88) -> (-18.844, 18.34) projected
  arc A38 (-20.528, 16.1347) -> (-18.844, 18.34) centre (-21.13, 18.34) ccw projected
  arc A39 (-23.416, 18.34) -> (-22.1, 16.27) centre (-21.13, 18.34) ccw projected
  line L101 (-23.416, 19.545) -> (-23.416, 20.88) projected
  point P0 (0, 0)
  dimension "d2" = 0.381
  dimension "d3" = 0.381
  dimension "d4" = 0.381
  dimension "d5" = 0.381
  dimension "d6" = 0.381
  dimension "d7" = 0.381
  dimension "d8" = 0.127
  constraints: 96 end point, 16 parallel, 8 perpendicular, 6 horizontal, 1 centre point, 18 other
  measures "d2" distance between parallel lines of L24 L75
  measures "d3" distance between parallel lines of L44 L79
  measures "d4" distance between parallel lines of L58 L86
  measures "d5" distance between parallel lines of L21 L90
  measures "d6" distance between parallel lines of L68 L91
  measures "d7" distance between parallel lines of L72 L95
  measures "d8" radial gap between concentric circles of A32 A37
extrude "Extrusion2" cut sketch "Sketch3" against normal blind 25.4 contours L8 A1 L26 A0 L42 L5 | L1 L31 A3 L30 A2 L4 | L42 A0 L26 A1 L8 L7 L6 L5 | L1 L2 L3 L4 A2 L30 A3 L31 | L42 A7 L41 A6 L13 L10 | L10 L11 L12 L13 A6 L41 A7 L42 | L17 A5 L37 A4 L36 L14 | L36 A4 L37 A5 L17 L16 L15 L14 | L18 A26 L21 | L18 A27 L19 A28 A29 A30 A31 A20 L20 A21 L21 A22 A23 A24 A25 A26 | L18 L19 A27 | A25 A24 L21 | L19 A29 A28 | A23 A22 L21 | L19 A31 A30 | A21 L20 L21 | L19 L20 A20 | L25 L24 L23 A38 L76 L75 L78 L77 A39 L22 | L22 A15 L25 | L22 A16 A17 A18 A19 L23 A38 A8 A9 L24 A10 A11 A12 A13 A14 L25 A15 | L22 A17 A16 | A14 L24 L25 | L22 A19 A18 | A13 A12 L24 | A39 L77 L76 A38 L23 L22 | A11 A10 L24 | L23 A8 A38 | A39 L43 L44 L45 L46 L101 L81 L80 | L80 L79 L82 L81 L101 L46 L45 L44 L43 A39 | A9 L23 L24 | L55 L56 L57 L58 | L67 L68 L69 L70 | L71 L72 L73 L74 | A32 | A33 | A34 | A35 | A36 | L83 L84 L85 L86 | L87 L88 L89 L90 | L94 L93 L92 L91 | L98 L97 L96 L95 | A37
sketch "Sketch4" plane through (0, 0, 3.175) normal (0, 0, 1) x (1, 0, 0)
  arc A0 (-19.989, 16.3591) -> (-18.844, 18.34) centre (-21.13, 18.34) ccw projected
  circle A1 centre (-21.13, 18.34) radius 1.5875
  arc A2 (-17.574, -29.92) -> (-22.146, -29.92) centre (-19.86, -29.92) ccw projected
  circle A3 centre (-19.86, -29.92) radius 1.5875
  arc A4 (-71.93, -27.126) -> (-71.93, -22.554) centre (-71.93, -24.84) ccw projected
  circle A5 centre (-71.93, -24.84) radius 1.5875
  arc A6 (-71.93, 0.814) -> (-71.93, 5.386) centre (-71.93, 3.1) ccw projected
  circle A7 centre (-71.93, 3.1) radius 1.5875
  line L0 (-73.5175, -34.0475) -> (-4.3025, -34.0475) projected
  line L1 (-4.3025, -34.0475) -> (-4.3025, 22.4675) projected
  line L2 (-4.3025, 22.4675) -> (-73.5175, 22.4675) projected
  line L3 (-73.5175, 22.4675) -> (-73.5175, 8.5836) projected
  line L4 (-73.5175, 8.5836) -> (-76.0575, 6.0436) projected
  line L5 (-76.0575, 6.0436) -> (-76.0575, -27.38) projected
  line L6 (-76.0575, -27.38) -> (-76.1056, -27.9894) projected
  line L7 (-76.1056, -27.9894) -> (-73.5175, -30.5776) projected
  line L8 (-73.5175, -30.5776) -> (-73.5175, -34.0475) projected
  line L9 (-28.371, 16.651) -> (-22.6705, 16.651) projected
  arc A8 (-23.035, 17.0764) -> (-22.6705, 16.651) centre (-21.13, 18.34) ccw projected
  line L10 (-23.035, 17.0764) -> (-23.035, 16.754) projected
  line L11 (-23.035, 16.754) -> (-49.197, 16.754) projected
  line L12 (-49.197, 16.754) -> (-49.197, 19.926) projected
  line L13 (-49.197, 19.926) -> (-23.416, 19.926) projected
  line L14 (-23.416, 19.926) -> (-23.416, 20.88) projected
  line L15 (-23.416, 20.88) -> (-18.844, 20.88) projected
  line L16 (-18.844, 20.88) -> (-18.844, 18.34) projected
  arc A9 (-19.989, 16.3591) -> (-18.844, 18.34) centre (-21.13, 18.34) ccw projected
  line L17 (-19.989, 16.3591) -> (-19.989, 10.889) projected
  line L18 (-19.989, 10.889) -> (-28.371, 10.889) projected
  line L19 (-28.371, 10.889) -> (-28.371, 16.651) projected
  line L20 (-32.179, -31.506) -> (-53.261, -31.506) projected
  line L21 (-53.261, -31.506) -> (-53.261, -28.334) projected
  line L22 (-53.261, -28.334) -> (-32.179, -28.334) projected
  line L23 (-32.179, -28.334) -> (-32.179, -31.506) projected
  circle A10 centre (-12.24, 16.943) radius 1.627 projected
  line L24 (-71.041, 19.926) -> (-49.959, 19.926) projected
  line L25 (-49.959, 19.926) -> (-49.959, 16.754) projected
  line L26 (-49.959, 16.754) -> (-71.041, 16.754) projected
  line L27 (-71.041, 16.754) -> (-71.041, 19.926) projected
  line L28 (-55.039, -31.506) -> (-71.041, -31.506) projected
  line L29 (-71.041, -31.506) -> (-71.041, -28.334) projected
  line L30 (-71.041, -28.334) -> (-55.039, -28.334) projected
  line L31 (-55.039, -28.334) -> (-55.039, -31.506) projected
  line L32 (-73.681, -8.761) -> (-73.681, -0.379) projected
  line L33 (-73.681, -0.379) -> (-67.919, -0.379) projected
  line L34 (-67.919, -0.379) -> (-67.919, -8.761) projected
  line L35 (-67.919, -8.761) -> (-73.681, -8.761) projected
  line L36 (-17.574, -32.46) -> (-22.146, -32.46) projected
  line L37 (-22.146, -32.46) -> (-22.146, -29.92) projected
  arc A11 (-17.574, -29.92) -> (-22.146, -29.92) centre (-19.86, -29.92) ccw projected
  line L38 (-17.574, -29.92) -> (-17.574, -32.46) projected
  line L39 (-74.47, 5.386) -> (-71.93, 5.386) projected
  arc A12 (-71.93, 0.814) -> (-71.93, 5.386) centre (-71.93, 3.1) ccw projected
  line L40 (-71.93, 0.814) -> (-74.47, 0.814) projected
  line L41 (-74.47, 0.814) -> (-74.47, 5.386) projected
  line L42 (-74.47, -27.126) -> (-74.47, -22.554) projected
  line L43 (-74.47, -22.554) -> (-71.93, -22.554) projected
  arc A13 (-71.93, -27.126) -> (-71.93, -22.554) centre (-71.93, -24.84) ccw projected
  line L44 (-71.93, -27.126) -> (-74.47, -27.126) projected
  line L45 (-22.6705, 16.651) -> (-19.989, 16.651)
  line L46 (-19.989, 16.651) -> (-19.989, 16.3591)
  line L47 (-19.989, 16.3591) -> (-22.6705, 16.651)
  line L48 (-23.035, 17.0764) -> (-23.416, 19.926)
  line L49 (-23.416, 19.926) -> (-23.035, 16.754)
  point P0 (0, 0)
  point P1 (-22.146, -29.92)
  point P2 (-71.93, 5.386)
  point P3 (-71.93, 0.814)
  dimension "d11" = 3.175
  dimension "d12" = 3.175
  dimension "d13" = 3.175
  dimension "d14" = 3.175
  constraints: 10 end point, 4 centre point, 4 coincident, 1 horizontal, 1 perpendicular
  measures "d11" diameter of A1
  measures "d12" diameter of A3
  measures "d13" diameter of A5
  measures "d14" diameter of A7
extrude "Extrusion3" add sketch "Sketch4" against normal blind 3.175 contours L46 L45 A8 L48 L14 L15 L16 A0 | L47 L45 L46 | L10 L49 L48 | L38 L36 L37 A2 | L44 L42 L43 A4 | L40 L41 L39 A6
sketch "Sketch6" plane through (0, 0, 3.175) normal (0, 0, 1) x (1, 0, 0)
  line L0 (-49.197, 19.926) -> (-23.416, 19.926) projected
  line L1 (-23.416, 19.926) -> (-23.416, 16.754)
  line L2 (-49.197, 16.754) -> (-23.035, 16.754) projected
  line L3 (-28.371, 16.651) -> (-22.6705, 16.651) projected
  line L4 (-23.416, 16.651) -> (-23.416, 16.3591)
  line L5 (-19.989, 16.3591) -> (-19.989, 10.889) projected
  line L6 (-23.416, 16.3591) -> (-19.989, 16.3591)
  circle A0 centre (-71.93, -24.84) radius 1.5875 projected
  circle A1 centre (-71.93, 3.1) radius 1.5875 projected
  circle A2 centre (-19.86, -29.92) radius 1.5875 projected
  line L7 (-19.989, 16.3591) -> (-19.989, 10.889) projected
  line L8 (-19.989, 10.889) -> (-28.371, 10.889) projected
  line L9 (-28.371, 10.889) -> (-28.371, 16.651) projected
  line L10 (-28.371, 16.651) -> (-22.6705, 16.651) projected
  line L11 (-22.6705, 16.651) -> (-19.989, 16.3591) projected
  circle A3 centre (-21.13, 18.34) radius 1.5875 projected
  line L12 (-73.5175, -34.0475) -> (-4.3025, -34.0475) projected
  line L13 (-4.3025, -34.0475) -> (-4.3025, 22.4675) projected
  line L14 (-4.3025, 22.4675) -> (-73.5175, 22.4675) projected
  line L15 (-73.5175, 22.4675) -> (-73.5175, 8.5836) projected
  line L16 (-73.5175, 8.5836) -> (-76.0575, 6.0436) projected
  line L17 (-76.0575, 6.0436) -> (-76.0575, -27.38) projected
  line L18 (-76.0575, -27.38) -> (-76.1056, -27.9894) projected
  line L19 (-76.1056, -27.9894) -> (-73.5175, -30.5776) projected
  line L20 (-73.5175, -30.5776) -> (-73.5175, -34.0475) projected
  line L21 (-23.416, 19.926) -> (-23.035, 16.754) projected
  line L22 (-23.035, 16.754) -> (-49.197, 16.754) projected
  line L23 (-49.197, 16.754) -> (-49.197, 19.926) projected
  line L24 (-49.197, 19.926) -> (-23.416, 19.926) projected
  line L25 (-32.179, -31.506) -> (-53.261, -31.506) projected
  line L26 (-53.261, -31.506) -> (-53.261, -28.334) projected
  line L27 (-53.261, -28.334) -> (-32.179, -28.334) projected
  line L28 (-32.179, -28.334) -> (-32.179, -31.506) projected
  circle A4 centre (-12.24, 16.943) radius 1.627 projected
  line L29 (-71.041, 19.926) -> (-49.959, 19.926) projected
  line L30 (-49.959, 19.926) -> (-49.959, 16.754) projected
  line L31 (-49.959, 16.754) -> (-71.041, 16.754) projected
  line L32 (-71.041, 16.754) -> (-71.041, 19.926) projected
  line L33 (-55.039, -31.506) -> (-71.041, -31.506) projected
  line L34 (-71.041, -31.506) -> (-71.041, -28.334) projected
  line L35 (-71.041, -28.334) -> (-55.039, -28.334) projected
  line L36 (-55.039, -28.334) -> (-55.039, -31.506) projected
  line L37 (-73.681, -8.761) -> (-73.681, -0.379) projected
  line L38 (-73.681, -0.379) -> (-67.919, -0.379) projected
  line L39 (-67.919, -0.379) -> (-67.919, -8.761) projected
  line L40 (-67.919, -8.761) -> (-73.681, -8.761) projected
  point P0 (0, 0)
  constraints: 6 end point, 4 point on line, 1 perpendicular, 1 vertical
extrude "Extrusion4" add sketch "Sketch6" against normal blind 3.175 contours L21 L2 L1 | L3 L11 L6 L4
sketch "Sketch7" plane through (0, 0, 3.175) normal (0, 0, 1) x (1, 0, 0)
  line L0 (-28.371, 16.651) -> (-23.416, 16.651) projected
  line L1 (-28.371, 16.651) -> (-23.416, 16.651)
  line L2 (-23.416, 16.651) -> (-23.416, 16.754)
  line L3 (-23.416, 16.754) -> (-28.371, 16.754)
  line L4 (-28.371, 16.754) -> (-28.371, 16.651)
  circle A0 centre (-71.93, -24.84) radius 1.5875 projected
  circle A1 centre (-71.93, 3.1) radius 1.5875 projected
  circle A2 centre (-19.86, -29.92) radius 1.5875 projected
  line L5 (-19.989, 16.3591) -> (-19.989, 10.889) projected
  line L6 (-19.989, 10.889) -> (-28.371, 10.889) projected
  line L7 (-28.371, 10.889) -> (-28.371, 16.651) projected
  line L8 (-28.371, 16.651) -> (-23.416, 16.651) projected
  line L9 (-23.416, 16.651) -> (-23.416, 16.3591) projected
  line L10 (-23.416, 16.3591) -> (-19.989, 16.3591) projected
  circle A3 centre (-21.13, 18.34) radius 1.5875 projected
  line L11 (-73.5175, -34.0475) -> (-4.3025, -34.0475) projected
  line L12 (-4.3025, -34.0475) -> (-4.3025, 22.4675) projected
  line L13 (-4.3025, 22.4675) -> (-73.5175, 22.4675) projected
  line L14 (-73.5175, 22.4675) -> (-73.5175, 8.5836) projected
  line L15 (-73.5175, 8.5836) -> (-76.0575, 6.0436) projected
  line L16 (-76.0575, 6.0436) -> (-76.0575, -27.38) projected
  line L17 (-76.0575, -27.38) -> (-76.1056, -27.9894) projected
  line L18 (-76.1056, -27.9894) -> (-73.5175, -30.5776) projected
  line L19 (-73.5175, -30.5776) -> (-73.5175, -34.0475) projected
  line L20 (-23.416, 16.754) -> (-49.197, 16.754) projected
  line L21 (-49.197, 16.754) -> (-49.197, 19.926) projected
  line L22 (-49.197, 19.926) -> (-23.416, 19.926) projected
  line L23 (-23.416, 19.926) -> (-23.416, 16.754) projected
  line L24 (-32.179, -31.506) -> (-53.261, -31.506) projected
  line L25 (-53.261, -31.506) -> (-53.261, -28.334) projected
  line L26 (-53.261, -28.334) -> (-32.179, -28.334) projected
  line L27 (-32.179, -28.334) -> (-32.179, -31.506) projected
  circle A4 centre (-12.24, 16.943) radius 1.627 projected
  line L28 (-71.041, 19.926) -> (-49.959, 19.926) projected
  line L29 (-49.959, 19.926) -> (-49.959, 16.754) projected
  line L30 (-49.959, 16.754) -> (-71.041, 16.754) projected
  line L31 (-71.041, 16.754) -> (-71.041, 19.926) projected
  line L32 (-55.039, -31.506) -> (-71.041, -31.506) projected
  line L33 (-71.041, -31.506) -> (-71.041, -28.334) projected
  line L34 (-71.041, -28.334) -> (-55.039, -28.334) projected
  line L35 (-55.039, -28.334) -> (-55.039, -31.506) projected
  line L36 (-73.681, -8.761) -> (-73.681, -0.379) projected
  line L37 (-73.681, -0.379) -> (-67.919, -0.379) projected
  line L38 (-67.919, -0.379) -> (-67.919, -8.761) projected
  line L39 (-67.919, -8.761) -> (-73.681, -8.761) projected
  point P0 (0, 0)
  constraints: 8 end point, 2 parallel, 1 horizontal, 1 perpendicular
extrude "Extrusion5" cut sketch "Sketch7" against normal blind 3.175 contours L4 L3 L2 L0
fillet "Fillet1" radius 1.6002 2 edges at (-28.371, 16.754, 1.5875) (-23.416, 16.3591, 1.5875)
sketch "Sketch8" plane through (0, 0, 3.175) normal (0, 0, 1) x (1, 0, 0)
  circle A0 centre (-12.24, 16.943) radius 1.627 projected
  circle A1 centre (-12.24, 16.943) radius 1.9714
  point P0 (0, 0)
  constraints: 1 centre point, 1 coincident
extrude "Extrusion6" cut sketch "Sketch8" against normal blind 25.4 contours A0 | A1
sketch "Sketch9" plane through (0, 0, 3.175) normal (0, 0, 1) x (1, 0, 0)
  line L0 (-23.416, 17.9593) -> (-23.416, 19.926) projected
  line L1 (-29.9712, 16.754) -> (-23.416, 16.754)
  line L2 (-23.416, 16.754) -> (-23.416, 19.926)
  line L3 (-23.416, 19.926) -> (-29.9712, 19.926)
  line L4 (-29.9712, 19.926) -> (-29.9712, 16.754)
  line L5 (-71.041, 19.926) -> (-71.041, 16.754) projected
  line L6 (-73.5175, 22.4675) -> (-4.3025, 22.4675) projected
  line L7 (-71.041, 19.926) -> (-23.416, 19.926)
  line L8 (-23.416, 19.926) -> (-23.416, 22.4675)
  line L9 (-23.416, 22.4675) -> (-71.041, 22.4675)
  line L10 (-71.041, 22.4675) -> (-71.041, 19.926)
  line L11 (-71.041, 19.926) -> (-29.9712, 19.926)
  line L12 (-29.9712, 19.926) -> (-29.9712, 16.754)
  line L13 (-29.9712, 16.754) -> (-71.041, 16.754)
  line L14 (-71.041, 16.754) -> (-71.041, 19.926)
  line L15 (-71.041, -31.506) -> (-55.039, -31.506) projected
  line L16 (-32.179, -31.506) -> (-32.179, -28.334) projected
  line L17 (-71.041, -31.506) -> (-32.179, -31.506)
  line L18 (-32.179, -31.506) -> (-32.179, -28.334)
  line L19 (-32.179, -28.334) -> (-71.041, -28.334)
  line L20 (-71.041, -28.334) -> (-71.041, -31.506)
  line L21 (-73.5175, -34.0475) -> (-4.3025, -34.0475) projected
  line L22 (-32.179, -31.506) -> (-71.041, -31.506)
  line L23 (-71.041, -31.506) -> (-71.041, -34.0475)
  line L24 (-71.041, -34.0475) -> (-32.179, -34.0475)
  line L25 (-32.179, -34.0475) -> (-32.179, -31.506)
  point P0 (0, 0)
  constraints: 40 end point, 10 parallel, 5 horizontal, 5 perpendicular, 3 point on line
extrude "Extrusion7" cut sketch "Sketch9" against normal blind 25.4
body "Solid1"
